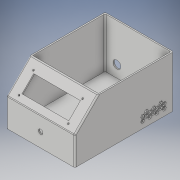
# Autodesk Inventor part: casenova
Saved by Autodesk Inventor 2019.4 (Build 234330000, 330)
## iProperties
Created: 2019-10-31
Part Number: casenova
Material: Genérico
Document SubType Name: Modeling
Designer: natha
Density: 1 g/cm^3
Appearance: Padrão
Author: natha
Autodesk Inventor part; units mm, degrees
ref_plane "YZ Plane" through (0, 0, 0) normal (1, 0, 0) x (0, 1, 0)
ref_plane "XZ Plane" through (0, 0, 0) normal (0, 1, 0) x (-1, 0, 0)
ref_plane "XY Plane" through (0, 0, 0) normal (0, 0, 1) x (1, 0, 0)
sketch "Esboço1" plane through (0, 0, 0) normal (0, 1, 0) x (-1, 0, 0)
  line L0 (-52, 75) -> (52, 75)
  line L1 (52, 75) -> (52, -75)
  line L2 (52, -75) -> (-52, -75)
  line L3 (-52, -75) -> (-52, 75)
  line L4 (-52, 75) -> (52, -75) construction
  line L5 (52, 75) -> (-52, -75) construction
  point P0 (0, 0)
  dimension "d0" = 104
  dimension "d1" = 150
  constraints: 12 end point, 2 midpoint, 2 parallel, 1 horizontal, 1 perpendicular
  measures "d0" distance of L1.end L2.end
  measures "d1" distance of L0.end L1.end
extrude "Extrusão1" add sketch "Esboço1" along normal blind 78
chamfer "Chanfro1" distance 35 angle 45 1 edges at (0, 78, 75) measured on face at (17.3333, 26, 75)
shell "Casca1" thickness 2 removed faces 1 at (-17.3333, 78, -36.6667)
sketch "Esboço2" plane through (-52, 78, 40) normal (0, 0.7071068, 0.7071068) x (1, 0, 0)
  line L0 (16.4, -39.4701) -> (87.6, -39.4701)
  line L1 (87.6, -39.4701) -> (87.6, -14.2701)
  line L2 (87.6, -14.2701) -> (16.4, -14.2701)
  line L3 (16.4, -14.2701) -> (16.4, -39.4701)
  line L4 (16.4, -39.4701) -> (87.6, -14.2701) construction
  line L5 (87.6, -39.4701) -> (16.4, -14.2701) construction
  point P0 (52, -26.8701)
  dimension "d8" = 25.2
  dimension "d9" = 71.2
  constraints: 12 end point, 2 midpoint, 2 parallel, 1 horizontal, 1 perpendicular
  measures "d8" distance of L0.end L1.end
  measures "d9" distance of L1.end L2.end
extrude "Extrusão2" cut sketch "Esboço2" against normal blind 5
sketch "Esboço6" plane through (52, 0, -75) normal (0, 0, -1) x (-1, 0, 0)
  line L0 (0, 0) -> (20, 0) construction
  line L1 (20, 14) -> (37.7, 14)
  line L2 (37.7, 14) -> (37.7, 25.1)
  line L3 (37.7, 25.1) -> (20, 25.1)
  line L4 (20, 25.1) -> (20, 14)
  line L5 (20, 0) -> (20, 14) construction
  line L6 (104, 0) -> (104, 43) construction
  line L7 (104, 0) -> (84, 0) construction
  line L8 (0, 0) -> (104, 0) construction
  line L9 (84, 0) -> (84, 20) construction
  circle A0 centre (84, 20) radius 6
  line L10 (20, 0) -> (20, 14)
  point P0 (52, 0)
  dimension "d34" = 20
  dimension "d36" = 14
  dimension "d37" = 20
  dimension "d38" = 20
  dimension "d39" = 12
  dimension "d42" = 17.7
  dimension "d43" = 11.1
  dimension "d117" = 14
  constraints: 18 end point, 3 equal length, 2 horizontal, 2 vertical, 1 centre point, 1 coincident, 1 perpendicular, 1 point on line
  measures "d34" distance of L0.start L0.end
  measures "d36" distance of L0.end L5.end
  measures "d37" distance of L6.start L7.end
  measures "d38" distance of L7.end L9.end
  measures "d39" diameter of A0
  measures "d42" distance of L2.end L3.end
  measures "d43" distance of L1.end L2.end
  measures "d117" distance of L0.end L5.end
extrude "Extrusão6" cut sketch "Esboço6" against normal blind 10
sketch "Esboço7" plane through (-52, 0, 75) normal (0, 0, 1) x (1, 0, 0)
  line L0 (87.6, 67.9095) -> (87.6, 50.0905) construction
  line L1 (16.4, 66.4953) -> (16.4, 48.6762) construction
  line L2 (104, 0) -> (0, 0) construction
  line L3 (0, 43) -> (104, 43) construction
  line L4 (104, 0) -> (104, 43) construction
  line L5 (104, 43) -> (104, 21.5) construction
  line L6 (104, 21.5) -> (0, 21.5) construction
  line L7 (0, 0) -> (0, 43) construction
  line L8 (87.6, 50.0905) -> (87.6, 21.5) construction
  line L9 (16.4, 48.439) -> (16.4, 21.5) construction
  circle A0 centre (52, 21.5) radius 3.5
  point P0 (52, 0)
  dimension "d48" = 43
  dimension "d49" = 71.2
  dimension "d50" = 7
  constraints: 8 end point, 3 midpoint, 3 point on line, 1 centre point, 1 perpendicular, 1 vertical
  measures "d48" distance between parallel lines of L2 L3
  measures "d49" distance between parallel lines of L9 L8
  measures "d50" diameter of A0
extrude "Extrusão8" cut sketch "Esboço7" against normal blind 10
sketch "Esboço13" plane through (-52, 78, 40) normal (0, 0.7071068, 0.7071068) x (1, 0, 0)
  line L0 (87.6, -14.2701) -> (87.6, -39.4701) projected
  line L1 (87.6, -39.4701) -> (16.4, -39.4701) projected
  line L2 (16.4, -39.4701) -> (16.4, -14.2701) projected
  line L3 (16.4, -14.2701) -> (87.6, -14.2701) projected
  line L4 (104, -49.4975) -> (104, 0) projected
  line L5 (104, 0) -> (0, 0) projected
  line L6 (0, 0) -> (0, -49.4975) projected
  line L7 (0, -49.4975) -> (104, -49.4975) projected
  line L8 (16.4, -14.2701) -> (87.6, -14.2701) construction
  line L9 (87.6, -14.2701) -> (87.6, -39.4701) construction
  line L10 (87.6, -39.4701) -> (16.4, -39.4701) construction
  line L11 (16.4, -39.4701) -> (16.4, -14.2701) construction
  line L12 (52, -26.8701) -> (11.45, -26.8701) construction
  line L13 (11.45, -26.8701) -> (11.45, -8.8701) construction
  line L14 (11.45, -8.8701) -> (11.45, -44.8701) construction
  line L15 (11.45, -44.8701) -> (91.45, -44.8701) construction
  line L16 (91.45, -44.8701) -> (91.45, -8.8701) construction
  line L17 (91.45, -8.8701) -> (11.45, -8.8701) construction
  line L18 (11.45, -44.8701) -> (13.95, -44.8701) construction
  line L19 (13.95, -44.8701) -> (13.95, -42.3701) construction
  line L20 (13.95, -42.3701) -> (11.45, -42.3701) construction
  line L21 (11.45, -42.3701) -> (11.45, -44.8701) construction
  line L22 (11.45, -8.8701) -> (13.95, -8.8701) construction
  line L23 (13.95, -8.8701) -> (13.95, -11.3701) construction
  line L24 (13.95, -11.3701) -> (11.45, -11.3701) construction
  line L25 (11.45, -11.3701) -> (11.45, -8.8701) construction
  line L26 (91.45, -8.8701) -> (88.95, -8.8701) construction
  line L27 (88.95, -8.8701) -> (88.95, -11.3701) construction
  line L28 (88.95, -11.3701) -> (91.45, -11.3701) construction
  line L29 (91.45, -11.3701) -> (91.45, -8.8701) construction
  line L30 (91.45, -44.8701) -> (88.95, -44.8701) construction
  line L31 (91.45, -42.3701) -> (91.45, -44.8701) construction
  line L32 (91.45, -44.8701) -> (88.95, -44.8701) construction
  line L33 (88.95, -44.8701) -> (88.95, -42.3701) construction
  line L34 (88.95, -42.3701) -> (91.45, -42.3701) construction
  line L35 (91.45, -42.3701) -> (91.45, -44.8701) construction
  circle A0 centre (88.95, -42.3701) radius 1.25
  circle A1 centre (88.95, -11.3701) radius 1.25
  circle A2 centre (13.95, -11.3701) radius 1.25
  circle A3 centre (13.95, -42.3701) radius 1.25
  dimension "d96" = 40.55
  dimension "d97" = 18
  dimension "d98" = 36
  dimension "d99" = 80
  dimension "d100" = 2.5
  dimension "d101" = 2.5
  dimension "d102" = 2.5
  dimension "d103" = 2.5
  dimension "d106" = 2.5
  dimension "d107" = 2.5
  dimension "d108" = 2.5
  dimension "d109" = 2.5
  dimension "d111" = 2.5
  dimension "d112" = 2.5
  dimension "d113" = 2.5
  dimension "d114" = 2.5
  constraints: 56 end point, 11 parallel, 8 perpendicular, 7 horizontal, 5 coincident, 4 centre point, 1 point on line
  measures "d96" distance of L12.start L12.end
  measures "d97" distance of L12.end L13.end
  measures "d98" distance of L13.end L14.end
  measures "d99" distance of L14.end L15.end
  measures "d100" distance of L20.end L19.end
  measures "d101" distance of L19.end L18.end
  measures "d102" distance of L23.end L24.end
  measures "d103" distance of L22.end L23.end
  measures "d106" distance of L26.end L27.end
  measures "d107" distance of L33.end L34.end
  measures "d108" distance of L32.end L33.end
  measures "d109" distance of L27.end L28.end
  measures "d111" diameter of A0
  measures "d112" diameter of A1
  measures "d113" diameter of A2
  measures "d114" diameter of A3
extrude "Extrusão12" cut sketch "Esboço13" against normal blind 10 contours A0 | A1 | A2 | A3
sketch "Esboço14" plane through (52, 0, 75) normal (1, 0, 0) x (0, 0, -1)
  line L0 (150, 0) -> (125, 0) construction
  line L1 (150, 0) -> (0, 0) construction
  line L2 (122.5, 18.7942) -> (121, 16.1962)
  line L3 (121, 16.1962) -> (118, 16.1962)
  line L4 (118, 16.1962) -> (116.5, 18.7942)
  line L5 (116.5, 18.7942) -> (118, 21.3923)
  line L6 (118, 21.3923) -> (121, 21.3923)
  line L7 (121, 21.3923) -> (122.5, 18.7942)
  line L8 (122.5, 12.5981) -> (121, 10)
  line L9 (121, 10) -> (118, 10)
  line L10 (118, 10) -> (116.5, 12.5981)
  line L11 (116.5, 12.5981) -> (118, 15.1962)
  line L12 (118, 15.1962) -> (121, 15.1962)
  line L13 (121, 15.1962) -> (122.5, 12.5981)
  line L14 (116.5, 12.5981) -> (115.5, 12.5981)
  line L15 (115.5, 12.5981) -> (115.5, 13.5981)
  line L16 (117, 16.1962) -> (115.5, 13.5981)
  line L17 (112.5, 13.5981) -> (111, 16.1962)
  line L18 (111, 16.1962) -> (112.5, 18.7942)
  line L19 (112.5, 18.7942) -> (115.5, 18.7942)
  line L20 (115.5, 18.7942) -> (117, 16.1962)
  line L21 (115.5, 13.5981) -> (112.5, 13.5981)
  line L22 (111.5, 19.7942) -> (110, 17.1962)
  line L23 (110, 17.1962) -> (107, 17.1962)
  line L24 (107, 17.1962) -> (105.5, 19.7942)
  line L25 (105.5, 19.7942) -> (107, 22.3923)
  line L26 (107, 22.3923) -> (110, 22.3923)
  line L27 (110, 22.3923) -> (111.5, 19.7942)
  line L28 (117, 10) -> (115.5, 7.4019)
  line L29 (115.5, 7.4019) -> (112.5, 7.4019)
  line L30 (112.5, 7.4019) -> (111, 10)
  line L31 (111, 10) -> (112.5, 12.5981)
  line L32 (112.5, 12.5981) -> (115.5, 12.5981)
  line L33 (115.5, 12.5981) -> (117, 10)
  line L34 (111.5, 13.5981) -> (110, 11)
  line L35 (107, 11) -> (105.5, 13.5981)
  line L36 (105.5, 13.5981) -> (107, 16.1962)
  line L37 (107, 16.1962) -> (110, 16.1962)
  line L38 (110, 16.1962) -> (111.5, 13.5981)
  line L39 (110, 11) -> (107, 11)
  line L40 (112.5, 13.5981) -> (112.5, 12.5981)
  line L41 (127.5, 19.7942) -> (129, 17.1962)
  line L42 (129, 22.3923) -> (127.5, 19.7942)
  line L43 (129, 17.1962) -> (132, 17.1962)
  line L44 (132, 17.1962) -> (133.5, 19.7942)
  line L45 (132, 22.3923) -> (129, 22.3923)
  line L46 (133.5, 19.7942) -> (132, 22.3923)
  line L47 (128, 16.1962) -> (126.5, 18.7942)
  line L48 (126.5, 13.5981) -> (128, 16.1962)
  line L49 (126.5, 18.7942) -> (123.5, 18.7942)
  line L50 (123.5, 18.7942) -> (122, 16.1962)
  line L51 (123.5, 13.5981) -> (126.5, 13.5981)
  line L52 (122, 16.1962) -> (123.5, 13.5981)
  line L53 (127.5, 13.5981) -> (129, 11)
  line L54 (129, 16.1962) -> (127.5, 13.5981)
  line L55 (129, 11) -> (132, 11)
  line L56 (132, 11) -> (133.5, 13.5981)
  line L57 (132, 16.1962) -> (129, 16.1962)
  line L58 (133.5, 13.5981) -> (132, 16.1962)
  line L59 (128, 10) -> (126.5, 12.5981)
  line L60 (126.5, 7.4019) -> (128, 10)
  line L61 (126.5, 12.5981) -> (123.5, 12.5981)
  line L62 (123.5, 12.5981) -> (122, 10)
  line L63 (122, 10) -> (123.5, 7.4019)
  line L64 (126.5, 7.4019) -> (123.5, 7.4019)
  line L65 (123.5, 12.5981) -> (122, 10)
  line L66 (123.5, 7.4019) -> (126.5, 7.4019)
  line L67 (126.5, 7.4019) -> (128, 10)
  line L68 (126.5, 12.5981) -> (123.5, 12.5981)
  line L69 (128, 10) -> (126.5, 12.5981)
  line L70 (122, 10) -> (123.5, 7.4019)
  line L71 (132, 16.1962) -> (133, 16.1962)
  line L72 (133, 16.1962) -> (134.5, 13.5981)
  line L73 (134.5, 18.7942) -> (133, 16.1962)
  line L74 (134.5, 13.5981) -> (137.5, 13.5981)
  line L75 (137.5, 18.7942) -> (134.5, 18.7942)
  line L76 (137.5, 13.5981) -> (139, 16.1962)
  line L77 (139, 16.1962) -> (137.5, 18.7942)
  line L78 (133, 10) -> (134.5, 7.4019)
  line L79 (137.5, 7.4019) -> (139, 10)
  line L80 (137.5, 12.5981) -> (134.5, 12.5981)
  line L81 (139, 10) -> (137.5, 12.5981)
  line L82 (134.5, 12.5981) -> (133, 10)
  line L83 (137.5, 7.4019) -> (134.5, 7.4019)
  line L84 (134.5, 12.5981) -> (133, 10)
  line L85 (133, 10) -> (134.5, 7.4019)
  line L86 (134.5, 7.4019) -> (137.5, 7.4019)
  line L87 (137.5, 7.4019) -> (139, 10)
  line L88 (137.5, 12.5981) -> (134.5, 12.5981)
  line L89 (139, 10) -> (137.5, 12.5981)
  line L90 (107, 16.1962) -> (106, 16.1962)
  line L91 (105.5, 12.5981) -> (104.5, 12.5981)
  line L92 (104.5, 12.5981) -> (104.5, 13.5981)
  line L93 (106, 16.1962) -> (104.5, 13.5981)
  line L94 (104.5, 18.7942) -> (106, 16.1962)
  line L95 (104.5, 13.5981) -> (101.5, 13.5981)
  line L96 (101.5, 13.5981) -> (100, 16.1962)
  line L97 (101.5, 18.7942) -> (104.5, 18.7942)
  line L98 (100, 16.1962) -> (101.5, 18.7942)
  line L99 (101.5, 13.5981) -> (101.5, 12.5981)
  line L100 (100, 10) -> (101.5, 12.5981)
  line L101 (101.5, 7.4019) -> (100, 10)
  line L102 (101.5, 12.5981) -> (104.5, 12.5981)
  line L103 (104.5, 12.5981) -> (106, 10)
  line L104 (104.5, 7.4019) -> (101.5, 7.4019)
  line L105 (106, 10) -> (104.5, 7.4019)
  line L106 (125, 0) -> (125, 10)
  point P0 (75, 0)
  point P1 (119.5, 18.7942)
  point P2 (119.5, 12.5981)
  point P3 (114, 16.1962)
  point P4 (108.5, 19.7942)
  point P5 (119.5, 11.2058)
  point P6 (108.5, 13.5981)
  point P7 (130.5, 19.7942)
  point P8 (125, 16.1962)
  point P9 (130.5, 13.5981)
  point P10 (130.5, 11.2058)
  point P11 (130.5, 11.2058)
  point P12 (136, 16.1962)
  point P13 (141.5, 11.2058)
  point P14 (141.5, 11.2058)
  point P15 (103, 16.1962)
  point P16 (108.5, 11.2058)
  dimension "d118" = 25
  dimension "d120" = 3
  dimension "d126" = 3
  dimension "d127" = 1
  dimension "d128" = 1
  dimension "d129" = 3
  dimension "d146" = 3
  dimension "d149" = 3
  dimension "d150" = 1
  dimension "d156" = 1
  dimension "d157" = 1
  dimension "d158" = 1
  dimension "d159" = 1
  dimension "d160" = 3
  dimension "d161" = 3
  dimension "d165" = 10
  constraints: 212 end point, 6 horizontal, 3 perpendicular, 1 point on line, 80 other
  measures "d118" distance of L0.start L0.end
  measures "d120" distance of L5.end L6.end
  measures "d126" distance of L11.end L12.end
  measures "d127" distance of L14.start L14.end
  measures "d128" distance of L14.end L15.end
  measures "d129" distance of L19.start L20.start
  measures "d146" distance of L40.end L32.end
  measures "d149" distance of L37.start L38.start
  measures "d150" distance of L34.start L40.start
  measures "d156" distance of L57.start L71.end
  measures "d157" distance of L37.start L90.end
  measures "d158" distance of L91.start L91.end
  measures "d159" distance of L91.end L92.end
  measures "d160" distance of L98.end L97.end
  measures "d161" distance of L102.start L103.start
  measures "d165" distance of L0.end L106.end
extrude "Extrusão14" cut sketch "Esboço14" against normal blind 10 contours L2 L3 L4 L5 L6 L7 | L8 L9 L10 L11 L12 L13 | L33 L28 L29 L30 L31 L32 | L21 L17 L18 L19 L20 L16 | L22 L23 L24 L25 L26 L27 | L34 L39 L35 L36 L37 L38 | L42 L45 L46 L44 L43 L41 | L48 L51 L52 L50 L49 L47 | L54 L57 L58 L56 L55 L53 | L60 L64 L63 L62 L61 L59 | L73 L75 L77 L76 L74 L72 | L82 L80 L81 L79 L83 L78 | L103 L105 L104 L101 L100 L102 | L95 L96 L98 L97 L94 L93
fillet "Arredondamento1" radius 2 9 edges at (-52, 39, -75) (-50, 40, -73) (50, 40, -73) (52, 39, -75) (-52, 21.5, 75) (-52, 60.5, 57.5) (0, 43, 75) (52, 21.5, 75) (52, 60.5, 57.5)
sketch "Esboço15" plane through (-50, 2, 73) normal (0, 1, 0) x (1, 0, 0)
  circle A0 centre (44.9013, 127.18) radius 1.8 projected
  circle A1 centre (54.9012, 127.2157) radius 1.8 projected
  circle A2 centre (45.124, 64.7844) radius 1.8 projected
  circle A3 centre (55.124, 64.8201) radius 1.8 projected
  point P0 (50, 73)
extrude "Extrusão15" cut sketch "Esboço15" against normal blind 10
